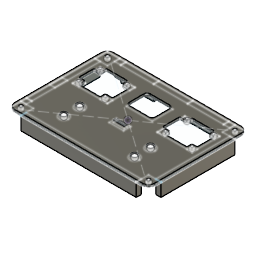
case cover (Autodesk Fusion 360 design; units mm, degrees)
part number: 2026-07-02-20-05-16-635
Autodesk Fusion 360 part; units mm, degrees
sketch "Sketch1" plane through (0, 0, 0) normal (0, 0, 1) x (1, 0, 0)
  line L0 (68, -48) -> (-68, -48)
  line L1 (-68, -48) -> (-68, 48)
  line L2 (-68, 48) -> (68, 48)
  line L3 (68, 48) -> (68, -48)
  line L4 (68, -48) -> (-68, 48) construction
  line L5 (-68, -48) -> (68, 48) construction
  line L6 (-68, 48) -> (-56, 48)
  line L7 (-56, 48) -> (-56, 36)
  line L8 (-56, 36) -> (-68, 36)
  line L9 (-68, 36) -> (-68, 48)
  line L10 (68, 48) -> (56, 48)
  line L11 (56, 48) -> (56, 36)
  line L12 (56, 36) -> (68, 36)
  line L13 (68, 36) -> (68, 48)
  line L14 (-68, -48) -> (-56, -48)
  line L15 (-56, -48) -> (-56, -36)
  line L16 (-56, -36) -> (-68, -36)
  line L17 (-68, -36) -> (-68, -48)
  line L18 (68, -48) -> (56, -48)
  line L19 (56, -48) -> (56, -36)
  line L20 (56, -36) -> (68, -36)
  line L21 (68, -36) -> (68, -48)
  circle A0 centre (-62, 42) radius 1.5
  circle A1 centre (62, 42) radius 1.5
  circle A2 centre (62, -42) radius 1.5
  circle A3 centre (-62, -42) radius 1.5
  line L22 (-56, 48) -> (-50, 48)
  line L23 (-50, 48) -> (-50, 43)
  line L24 (-50, 43) -> (-56, 43)
  line L25 (-56, 43) -> (-56, 48)
  line L26 (56, 48) -> (50, 48)
  line L27 (50, 48) -> (50, 43)
  line L28 (50, 43) -> (56, 43)
  line L29 (56, 43) -> (56, 48)
  line L30 (68, 36) -> (63, 36)
  line L31 (63, 36) -> (63, -36)
  line L32 (63, -36) -> (68, -36)
  line L33 (68, -36) -> (68, 36)
  line L34 (-68, 36) -> (-63, 36)
  line L35 (-63, 36) -> (-63, -30.6)
  line L36 (-63, -30.6) -> (-68, -30.6)
  line L37 (-68, -30.6) -> (-68, 36)
  line L38 (-63, -30.6) -> (-68, -30.6)
  line L39 (-68, -30.6) -> (-68, -36)
  line L40 (-68, -36) -> (-63, -36)
  line L41 (-63, -36) -> (-63, -30.6)
  line L42 (56, -48) -> (-56, -48)
  line L43 (-56, -48) -> (-56, -43)
  line L44 (-56, -43) -> (56, -43)
  line L45 (56, -43) -> (56, -48)
  line L46 (-5.3, -6) -> (5.3, -6)
  line L47 (5.3, -6) -> (5.3, -9)
  line L48 (5.3, -9) -> (-5.3, -9)
  line L49 (-5.3, -9) -> (-5.3, -6)
  circle A4 centre (-34.4, -28) radius 3
  circle A5 centre (-34.4, -12.5) radius 3
  circle A6 centre (34.4, -28) radius 3
  circle A7 centre (34.4, -12.5) radius 3
  line L50 (-12.5, 31) -> (12.5, 31)
  line L51 (12.5, 31) -> (12.5, 11)
  line L52 (12.5, 11) -> (-12.5, 11)
  line L53 (-12.5, 11) -> (-12.5, 31)
  line L54 (24.3, 31) -> (58, 31)
  line L55 (58, 31) -> (58, 4.3)
  line L56 (58, 4.3) -> (24.3, 4.3)
  line L57 (24.3, 4.3) -> (24.3, 31)
  line L58 (-58, 31) -> (-24.3, 31)
  line L59 (-24.3, 31) -> (-24.3, 4.3)
  line L60 (-24.3, 4.3) -> (-58, 4.3)
  line L61 (-58, 4.3) -> (-58, 31)
  circle A8 centre (-29.3, 28) radius 1.3
  circle A9 centre (-29.3, 7.3) radius 1.3
  circle A10 centre (-55, 7.3) radius 1.3
  circle A11 centre (-55, 28) radius 1.3
  line L62 (-58, 31) -> (-52, 31)
  line L63 (-52, 31) -> (-52, 25)
  line L64 (-52, 25) -> (-58, 25)
  line L65 (-58, 25) -> (-58, 31)
  line L66 (-58, 4.3) -> (-52, 4.3)
  line L67 (-52, 4.3) -> (-52, 10.3)
  line L68 (-52, 10.3) -> (-58, 10.3)
  line L69 (-58, 10.3) -> (-58, 4.3)
  line L70 (-24.3, 31) -> (-31.3, 31)
  line L71 (-31.3, 31) -> (-31.3, 26)
  line L72 (-31.3, 26) -> (-24.3, 26)
  line L73 (-24.3, 26) -> (-24.3, 31)
  line L74 (-24.3, 4.3) -> (-31.3, 4.3)
  line L75 (-31.3, 4.3) -> (-31.3, 9.3)
  line L76 (-31.3, 9.3) -> (-24.3, 9.3)
  line L77 (-24.3, 9.3) -> (-24.3, 4.3)
  line L78 (-7.3, -4) -> (6.7, -4)
  line L79 (6.7, -4) -> (6.7, -11)
  line L80 (6.7, -11) -> (-7.3, -11)
  line L81 (-7.3, -11) -> (-7.3, -4)
  circle A12 centre (29.3, 28) radius 1.3
  circle A13 centre (29.3, 7.3) radius 1.3
  circle A14 centre (55, 28) radius 1.3
  circle A15 centre (55, 7.3) radius 1.3
  line L82 (58, 31) -> (53, 31)
  line L83 (53, 31) -> (53, 26)
  line L84 (53, 26) -> (58, 26)
  line L85 (58, 26) -> (58, 31)
  line L86 (58, 4.3) -> (53, 4.3)
  line L87 (53, 4.3) -> (53, 9.3)
  line L88 (53, 9.3) -> (58, 9.3)
  line L89 (58, 9.3) -> (58, 4.3)
  line L90 (24.3, 4.3) -> (31.3, 4.3)
  line L91 (31.3, 4.3) -> (31.3, 9.3)
  line L92 (31.3, 9.3) -> (24.3, 9.3)
  line L93 (24.3, 9.3) -> (24.3, 4.3)
  line L94 (24.3, 31) -> (31.3, 31)
  line L95 (31.3, 31) -> (31.3, 26)
  line L96 (31.3, 26) -> (24.3, 26)
  line L97 (24.3, 26) -> (24.3, 31)
  line L98 (-50, 48) -> (-18, 48)
  line L99 (-18, 48) -> (-18, 43)
  line L100 (-18, 43) -> (-50, 43)
  line L101 (-50, 43) -> (-50, 48)
  line L102 (50, 48) -> (15, 48)
  line L103 (15, 48) -> (15, 43)
  line L104 (15, 43) -> (50, 43)
  line L105 (50, 43) -> (50, 48)
  circle A16 centre (-34.4, -12.5) radius 4.5
  circle A17 centre (-34.4, -28) radius 4.5
  circle A18 centre (34.4, -28) radius 4.5
  circle A19 centre (34.4, -12.5) radius 4.5
  line L106 (-68, 4) -> (-63, 4)
  line L107 (-63, 4) -> (-63, -8)
  line L108 (-63, -8) -> (-68, -8)
  line L109 (-68, -8) -> (-68, 4)
  line L110 (15, 48) -> (-18, 48)
  line L111 (-18, 48) -> (-18, 43)
  line L112 (-18, 43) -> (15, 43)
  line L113 (15, 43) -> (15, 48)
  dimension "d1" = 136
  dimension "d2" = 96
  dimension "d3" = 12
  dimension "d4" = 12
  dimension "d5" = 12
  dimension "d6" = 12
  dimension "d7" = 12
  dimension "d8" = 12
  dimension "d9" = 12
  dimension "d10" = 12
  dimension "d11" = 3
  dimension "d12" = 6
  dimension "d13" = 6
  dimension "d14" = 3
  dimension "d15" = 3
  dimension "d16" = 3
  dimension "d17" = 6
  dimension "d18" = 6
  dimension "d19" = 6
  dimension "d20" = 6
  dimension "d21" = 6
  dimension "d22" = 6
  dimension "d23" = 6
  dimension "d24" = 5
  dimension "d25" = 6
  dimension "d26" = 5
  dimension "d27" = 5
  dimension "d28" = 5
  dimension "d29" = 66.6
  dimension "d30" = 5
  dimension "d31" = 10.6
  dimension "d32" = 3
  dimension "d33" = 5.3
  dimension "d34" = 34
  dimension "d35" = 6
  dimension "d36" = 6
  dimension "d37" = 6
  dimension "d38" = 6
  dimension "d39" = 15
  dimension "d40" = 28.6
  dimension "d41" = 28.6
  dimension "d42" = 30.5
  dimension "d43" = 28.6
  dimension "d44" = 28.6
  dimension "d45" = 15
  dimension "d46" = 30.5
  dimension "d47" = 25
  dimension "d48" = 20
  dimension "d49" = 12.5
  dimension "d51" = 5
  dimension "d52" = 33.7
  dimension "d53" = 26.7
  dimension "d54" = 5
  dimension "d55" = 5
  dimension "d56" = 33.7
  dimension "d57" = 26.7
  dimension "d58" = 5
  dimension "d59" = 5
  dimension "d60" = 2.6
  dimension "d61" = 3
  dimension "d62" = 5
  dimension "d63" = 2.6
  dimension "d64" = 2.6
  dimension "d65" = 2.6
  dimension "d66" = 5
  dimension "d67" = 3
  dimension "d68" = 3
  dimension "d69" = 3
  dimension "d70" = 3
  dimension "d71" = 3
  dimension "d72" = 6
  dimension "d73" = 6
  dimension "d74" = 6
  dimension "d75" = 6
  dimension "d76" = 7
  dimension "d77" = 5
  dimension "d78" = 7
  dimension "d79" = 5
  dimension "d80" = 14
  dimension "d81" = 7
  dimension "d82" = 2
  dimension "d83" = 2
  dimension "d84" = 2.6
  dimension "d85" = 2.6
  dimension "d86" = 2.6
  dimension "d87" = 2.6
  dimension "d88" = 3
  dimension "d89" = 5
  dimension "d90" = 5
  dimension "d91" = 3
  dimension "d92" = 3
  dimension "d93" = 3
  dimension "d94" = 3
  dimension "d95" = 3
  dimension "d96" = 5
  dimension "d97" = 5
  dimension "d98" = 5
  dimension "d99" = 5
  dimension "d100" = 7
  dimension "d101" = 5
  dimension "d102" = 7
  dimension "d103" = 5
  dimension "d104" = 32
  dimension "d105" = 5
  dimension "d106" = 35
  dimension "d107" = 5
  dimension "d124" = 9
  dimension "d125" = 9
  dimension "d126" = 9
  dimension "d127" = 9
  dimension "d134" = 28
  dimension "d135" = 12
  constraint horizontal L0
  constraint perpendicular L0 L1
  constraint parallel L0 L2
  constraint parallel L1 L3
  constraint coincident L4 origin
  constraint coincident L5 origin
  constraint horizontal L6
  constraint vertical L7
  constraint horizontal L8
  constraint vertical L9
  constraint horizontal L10
  constraint vertical L11
  constraint horizontal L12
  constraint vertical L13
  constraint horizontal L14
  constraint vertical L15
  constraint horizontal L16
  constraint vertical L17
  constraint horizontal L18
  constraint vertical L19
  constraint horizontal L20
  constraint vertical L21
  constraint horizontal L22
  constraint vertical L23
  constraint horizontal L24
  constraint vertical L25
  constraint horizontal L26
  constraint vertical L27
  constraint horizontal L28
  constraint vertical L29
  constraint horizontal L30
  constraint vertical L31
  constraint horizontal L32
  constraint vertical L33
  constraint horizontal L34
  constraint vertical L35
  constraint horizontal L36
  constraint vertical L37
  constraint horizontal L38
  constraint vertical L39
  constraint horizontal L40
  constraint vertical L41
  constraint horizontal L42
  constraint vertical L43
  constraint horizontal L44
  constraint vertical L45
  constraint horizontal L46
  constraint vertical L47
  constraint horizontal L48
  constraint vertical L49
  constraint horizontal L50
  constraint vertical L51
  constraint horizontal L52
  constraint vertical L53
  constraint horizontal L54
  constraint vertical L55
  constraint horizontal L56
  constraint vertical L57
  constraint horizontal L58
  constraint vertical L59
  constraint horizontal L60
  constraint vertical L61
  constraint horizontal L62
  constraint vertical L63
  constraint horizontal L64
  constraint vertical L65
  constraint horizontal L66
  constraint vertical L67
  constraint horizontal L68
  constraint vertical L69
  constraint horizontal L70
  constraint vertical L71
  constraint horizontal L72
  constraint vertical L73
  constraint horizontal L74
  constraint vertical L75
  constraint horizontal L76
  constraint vertical L77
  constraint horizontal L78
  constraint vertical L79
  constraint horizontal L80
  constraint vertical L81
  constraint horizontal L82
  constraint vertical L83
  constraint horizontal L84
  constraint vertical L85
  constraint horizontal L86
  constraint vertical L87
  constraint horizontal L88
  constraint vertical L89
  constraint horizontal L90
  constraint vertical L91
  constraint horizontal L92
  constraint vertical L93
  constraint horizontal L94
  constraint vertical L95
  constraint horizontal L96
  constraint vertical L97
  constraint horizontal L98
  constraint vertical L99
  constraint horizontal L100
  constraint vertical L101
  constraint horizontal L102
  constraint vertical L103
  constraint horizontal L104
  constraint vertical L105
  constraint concentric A5 A16
  constraint concentric A4 A17
  constraint concentric A6 A18
  constraint concentric A7 A19
  constraint horizontal L106
  constraint vertical L107
  constraint horizontal L108
  constraint vertical L109
  constraint coincident L35 L107.end
  constraint coincident L1 L106.start
  constraint horizontal L110
  constraint vertical L111
  constraint horizontal L112
  constraint vertical L113
  measures "d1" distance of L1.end L2.end
  measures "d2" distance of L0.end L1.end
  measures "d3" distance of L1.end L6.end
  measures "d4" distance of L1.end L8.end
  measures "d5" distance of L2.end L10.end
  measures "d6" distance of L2.end L12.end
  measures "d7" distance of L0.end L14.end
  measures "d8" distance of L0.end L16.end
  measures "d9" distance of L0.start L18.end
  measures "d10" distance of L0.start L20.end
  measures "d11" diameter of A0
  measures "d12" distance of L2 A0.centre
  measures "d13" distance of L1 A0.centre
  measures "d14" diameter of A1
  measures "d15" diameter of A2
  measures "d16" diameter of A3
  measures "d17" distance of L2 A1.centre
  measures "d18" distance of L13 A1.centre
  measures "d19" distance of L21 A2.centre
  measures "d20" distance of L0 A2.centre
  measures "d21" distance of L16 A3.centre
  measures "d22" distance of L17 A3.centre
  measures "d23" distance of L6.end L22.end
  measures "d24" distance of L6.end L24.end
  measures "d25" distance of L10.end L26.end
  measures "d26" distance of L10.end L28.end
  measures "d27" distance of L12.end L30.end
  measures "d28" distance of L8.end L34.end
  measures "d29" distance of L8.end L36.end
  measures "d30" distance of L18.end L44.end
  measures "d31" distance of L46.start L46.end
  measures "d32" distance of L46.start L48.end
  measures "d33" distance of origin L49
  measures "d34" distance of L44 L48
  measures "d35" diameter of A4
  measures "d36" diameter of A5
  measures "d37" diameter of A6
  measures "d38" diameter of A7
  measures "d39" distance of L44 A4.centre
  measures "d40" distance of L35 A4.centre
  measures "d41" distance of L35 A5.centre
  measures "d42" distance of L44 A5.centre
  measures "d43" distance of L31 A7.centre
  measures "d44" distance of L31 A6.centre
  measures "d45" distance of L44 A6.centre
  measures "d46" distance of L44 A7.centre
  measures "d47" distance of L50.start L50.end
  measures "d48" distance of L50.start L52.end
  measures "d49" distance of origin L51
  measures "d51" distance of L12 L50
  measures "d52" distance of L54.start L54.end
  measures "d53" distance of L54.start L56.end
  measures "d54" distance of L12 L54
  measures "d55" distance of L31 L55
  measures "d56" distance of L58.start L58.end
  measures "d57" distance of L58.start L60.end
  measures "d58" distance of L8 L58
  measures "d59" distance of L35 L61
  measures "d60" diameter of A8
  measures "d61" distance of L58 A8.centre
  measures "d62" distance of L59 A8.centre
  measures "d63" diameter of A9
  measures "d64" diameter of A10
  measures "d65" diameter of A11
  measures "d66" distance of L59 A9.centre
  measures "d67" distance of L60 A9.centre
  measures "d68" distance of L60 A10.centre
  measures "d69" distance of L61 A10.centre
  measures "d70" distance of L58 A11.centre
  measures "d71" distance of L61 A11.centre
  measures "d72" distance of L58.start L62.end
  measures "d73" distance of L58.start L64.end
  measures "d74" distance of L60.end L66.end
  measures "d75" distance of L60.end L68.end
  measures "d76" distance of L58.end L70.end
  measures "d77" distance of L58.end L72.end
  measures "d78" distance of L59.end L74.end
  measures "d79" distance of L59.end L76.end
  measures "d80" distance of L78.start L78.end
  measures "d81" distance of L78.start L80.end
  measures "d82" distance of L49 L81
  measures "d83" distance of L48 L80
  measures "d84" diameter of A12
  measures "d85" diameter of A13
  measures "d86" diameter of A14
  measures "d87" diameter of A15
  measures "d88" distance of L54 A12.centre
  measures "d89" distance of L57 A12.centre
  measures "d90" distance of L57 A13.centre
  measures "d91" distance of L56 A13.centre
  measures "d92" distance of L55 A15.centre
  measures "d93" distance of L56 A15.centre
  measures "d94" distance of L54 A14.centre
  measures "d95" distance of L55 A14.centre
  measures "d96" distance of L54.end L82.end
  measures "d97" distance of L54.end L84.end
  measures "d98" distance of L55.end L86.end
  measures "d99" distance of L55.end L88.end
  measures "d100" distance of L56.end L90.end
  measures "d101" distance of L56.end L92.end
  measures "d102" distance of L54.start L94.end
  measures "d103" distance of L54.start L96.end
  measures "d104" distance of L22.end L98.end
  measures "d105" distance of L22.end L23.end
  measures "d106" distance of L26.end L102.end
  measures "d107" distance of L26.end L27.end
  measures "d124" diameter of A16
  measures "d125" diameter of A17
  measures "d126" diameter of A18
  measures "d127" diameter of A19
  measures "d134" distance of L40 L108
  measures "d135" distance of L106 L108
extrude "Extrude1" add sketch "Sketch1" along normal blind 2 contours L0 L3 L18 L19 L20 L21 L32 L45 | L0 L15 L19 L42 L43 L44 L45 | L3 L12 L20 L30 L31 L32 L33 | L0 L1 L14 L15 L16 L17 L40 L43 | L7 L8 L11 L12 L15 L16 L19 L20 L24 L28 L31 L35 L41 L44 L100 L104 L107 L112 | L2 L3 L10 L11 L12 L13 L29 L30 | L1 L16 L36 L38 L39 L40 L41 | L2 L11 L26 L27 L28 L29 L105 | L1 L35 L36 L37 L38 L108 | L2 L27 L102 L103 L104 L105 L113 | L1 L35 L37 L106 L107 L108 L109 | L2 L99 L103 L110 L111 L112 L113 | L1 L8 L34 L35 L37 L106 | L2 L23 L98 L99 L100 L101 L111 | L1 L2 L6 L7 L8 L9 L25 L34 | L2 L7 L22 L23 L24 L25 L101 | L54 L57 L94 L95 L96 L97 | L54 L55 L82 L83 L84 L85 | L56 L57 L90 L91 L92 L93 | L55 L56 L86 L87 L88 L89 | L58 L61 L62 L63 L64 L65 | L58 L59 L70 L71 L72 L73 | L60 L61 L66 L67 L68 L69 | L59 L60 L74 L75 L76 L77 | L78 L79 L80 L81 | A16 | A17 | A18 | A19 makes body 1
fillet "Fillet1" radius 6 4 edges at (68, -48, 1) (-68, -48, 1) (68, 48, 1) (-68, 48, 1) on bodies 1
fillet "Fillet2" radius 3 4 edges at (12.5, 31, 1) (-12.5, 31, 1) (-12.5, 11, 1) (12.5, 11, 1) on bodies 1
fillet "Fillet3" radius 1 4 edges at (-52, 25, 1) (-31.3, 26, 1) (-31.3, 9.3, 1) (-52, 10.3, 1) on bodies 1
fillet "Fillet4" radius 1 4 edges at (31.3, 26, 1) (53, 26, 1) (53, 9.3, 1) (31.3, 9.3, 1) on bodies 1
fillet "Fillet5" radius 1 6 edges at (-52, 31, 1) (-31.3, 31, 1) (-24.3, 26, 1) (-24.3, 9.3, 1) (-31.3, 4.3, 1) (-52, 4.3, 1) on bodies 1
fillet "Fillet6" radius 1 2 edges at (-58, 10.3, 1) (-58, 25, 1) on bodies 1
fillet "Fillet7" radius 1 8 edges at (53, 31, 1) (31.3, 31, 1) (31.3, 4.3, 1) (53, 4.3, 1) (58, 9.3, 1) (58, 26, 1) (24.3, 26, 1) (24.3, 9.3, 1) on bodies 1
extrude "Extrude2" add sketch "Sketch1" against normal blind 7 separate body contours A16 | A17 | A18 | A19 makes body 2 at (38.8776, -12.9481, -4.6667) makes body 3 at (38.8776, -28.4481, -4.6667) makes body 4 at (-29.9224, -12.9481, -4.6667) makes body 5 at (-29.9224, -28.4481, -4.6667)
extrude "Extrude3" add sketch "Sketch1" against normal blind 7 separate body contours L78 L79 L80 L81 makes body 6
fillet "Fillet8" radius 1 4 edges at (6.7, -11, -3.5) (6.7, -4, -3.5) (-7.3, -11, -3.5) (-7.3, -4, -3.5) on bodies 6
extrude "Extrude4" add sketch "Sketch1" against normal blind 13 separate body contours L0 L15 L19 L42 L43 L44 L45 | L3 L12 L20 L30 L31 L32 L33 | L2 L11 L26 L27 L28 L29 L105 | L1 L35 L36 L37 L38 L108 | L1 L8 L34 L35 L37 L106 | L2 L7 L22 L23 L24 L25 L101 makes body 7 at (52, 43, -4.3333) makes body 8 at (-68, -23.0667, -4.3333) makes body 9 at (63, 12, -4.3333) makes body 10 at (-52, 43, -4.3333) makes body 11 at (-68, 14.6667, -8.6667) makes body 12 at (-18.6667, -43, -4.3333)
extrude "Extrude5" add sketch "Sketch1" against normal blind 2 contours L1 L16 L36 L38 L39 L40 L41 | L1 L35 L37 L106 L107 L108 L109 bodies 1 8 11
extrude "Extrude6" add sketch "Sketch1" against normal blind 15 contours L2 L27 L102 L103 L104 L105 L113 bodies 1 7
extrude "Extrude7" add sketch "Sketch1" against normal blind 15 contours L2 L23 L98 L99 L100 L101 L111 bodies 1 10
extrude "Extrude8" add sketch "Sketch1" against normal blind 11 contours L2 L99 L103 L110 L111 L112 L113 bodies 1
fillet "Fillet9" radius 2 2 edges at (15, 45.5, -11) (-18, 45.5, -11) on bodies 1
equation "d29 = 72 mm - 5.4 mm"
